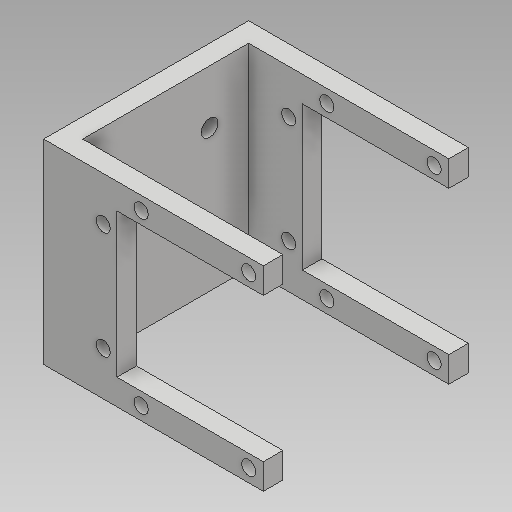
# Autodesk Inventor part: connection_hand
Saved by Autodesk Inventor 2017 (Build 210142000, 142)
## iProperties
Part Number: connection_hand
Material: Aluminium 6061
Document SubType Name: Modeling
Designer: Max
Density: 2.7 g/cm^3
Appearance: Vorgabe
Mass: 33.2037 g
Surface Area: 85.4905 cm^2
Volume: 12.2977 cm^3
Author: Max
Autodesk Inventor part; units mm, degrees
ref_plane "YZ Plane" through (0, 0, 0) normal (1, 0, 0) x (0, 1, 0)
ref_plane "XZ Plane" through (0, 0, 0) normal (0, 1, 0) x (-1, 0, 0)
ref_plane "XY Plane" through (0, 0, 0) normal (0, 0, 1) x (1, 0, 0)
sketch "Skizze1" plane through (0, 0, 0) normal (1, 0, 0) x (0, 1, 0)
  line L0 (-21, 20) -> (21, 20)
  line L1 (21, 20) -> (21, -20)
  line L2 (21, -20) -> (-21, -20)
  line L3 (-21, -20) -> (-21, 20)
  line L4 (-21, 20) -> (21, -20) construction
  line L5 (21, 20) -> (-21, -20) construction
  point P0 (0, 0)
  dimension "d0" = 42
  dimension "d1" = 40
  constraints: 12 end point, 2 midpoint, 2 parallel, 1 horizontal, 1 perpendicular
  measures "d0" distance of L1.end L2.end
  measures "d1" distance of L0.end L1.end
extrude "Extrusion1" add sketch "Skizze1" along normal blind 45
sketch "Skizze2" plane through (0, -21, 20) normal (0, 0, 1) x (1, 0, 0)
  line L0 (0, 0) -> (0, 42) projected
  line L1 (0, 0) -> (45, 0) projected
  line L2 (45, 42) -> (45, 0) projected
  line L3 (0, 42) -> (45, 42) projected
  line L4 (45, 42) -> (45, 0) projected
  line L5 (45, 38) -> (4, 38)
  line L6 (4, 38) -> (4, 4)
  line L7 (4, 4) -> (45, 4)
  line L8 (45, 4) -> (45, 38)
  point P0 (0, 21)
  dimension "d4" = 4
  dimension "d5" = 4
  dimension "d6" = 4
  constraints: 8 end point, 2 parallel, 1 horizontal, 1 perpendicular, 1 point on line
  measures "d4" distance between parallel lines of L5 L3
  measures "d5" distance between parallel lines of L1 L7
  measures "d6" distance between parallel lines of L0 L6
extrude "Extrusion2" cut sketch "Skizze2" against normal through all contours L7 L6 L5 L2
sketch "Skizze3" plane through (0, -21, -20) normal (0, -1, 0) x (1, 0, 0)
  line L0 (0, 0) -> (0, 40) projected
  line L1 (0, 0) -> (45, 0) projected
  line L2 (45, 40) -> (45, 0) projected
  line L3 (0, 40) -> (45, 40) projected
  line L4 (0, 20) -> (44.7617, 20) construction
  line L5 (15, 34.75) -> (45, 34.75)
  line L6 (45, 34.75) -> (45, 5.25)
  line L7 (45, 5.25) -> (15, 5.25)
  line L8 (15, 5.25) -> (15, 34.75)
  line L9 (15, 34.75) -> (45, 5.25) construction
  line L10 (45, 34.75) -> (15, 5.25) construction
  point P0 (30, 20)
  dimension "d9" = 29.5
  dimension "d10" = 30
  constraints: 14 end point, 2 horizontal, 2 midpoint, 2 parallel, 2 point on line, 1 perpendicular
  measures "d9" distance of L7.end L5.start
  measures "d10" distance of L6.end L7.end
extrude "Extrusion3" cut sketch "Skizze3" against normal through all contours L7 L8 L5 L2
sketch "Skizze4" plane through (0, -21, -20) normal (0, -1, 0) x (1, 0, 0)
  line L0 (45, 5.25) -> (15, 5.25) projected
  line L1 (15, 5.25) -> (15, 34.75) projected
  line L2 (15, 34.75) -> (45, 34.75) projected
  line L3 (45, 40) -> (45, 34.75) projected
  line L4 (0, 40) -> (45, 40) projected
  line L5 (0, 0) -> (0, 40) projected
  line L6 (0, 0) -> (45, 0) projected
  line L7 (45, 5.25) -> (45, 0) projected
  line L8 (0, 20) -> (84.4351, 20) construction
  point P0 (20, 37.3)
  point P1 (20, 2.7)
  point P2 (12.2, 31)
  point P3 (12.2, 9)
  point P4 (42, 37.3)
  point P5 (42, 2.7)
  dimension "d13" = 5
  dimension "d14" = 5
  dimension "d15" = 34.6
  dimension "d16" = 17.3
  dimension "d17" = 22
  dimension "d18" = 11
  dimension "d19" = 2.8
  dimension "d20" = 2.8
  dimension "d47" = 17.3
  dimension "d48" = 17.3
  dimension "d49" = 22
  dimension "d50" = 22
  constraints: 2 end point, 1 horizontal
  measures "d13" distance from line of point (20, 2.7) L1
  measures "d14" distance from line of L1 point (20, 37.3)
  measures "d15" distance of point (20, 2.7) point (20, 37.3)
  measures "d16" distance from line of L8 point (20, 37.3)
  measures "d17" distance of point (12.2, 9) point (12.2, 31)
  measures "d18" distance from line of L8 point (12.2, 31)
  measures "d19" distance from line of L1 point (12.2, 31)
  measures "d20" distance from line of L1 point (12.2, 9)
  measures "d47" distance from line of point (42, 37.3) L8
  measures "d48" distance from line of L8 point (42, 2.7)
  measures "d49" distance of point (42, 37.3) point (20, 37.3)
  measures "d50" distance of point (42, 2.7) point (20, 2.7)
hole "Bohrung1" at (20, -21, 17.3) at (20, -21, -17.3) at (12.2, -21, 11) at (12.2, -21, -11) at (42, -21, 17.3) at (42, -21, -17.3) direction (0, 1, 0) diameter 2.9 end through all clearance for "Inbusschraube ISO 4762" size "M2.5" standard "ISO"
sketch "Skizze7" plane through (4, -17, 20) normal (1, 0, 0) x (0, 0, -1)
  line L0 (29, 8) -> (11, 8)
  line L1 (11, 8) -> (11, 26)
  line L2 (11, 26) -> (29, 26)
  line L3 (29, 26) -> (29, 8)
  line L4 (29, 8) -> (11, 26) construction
  line L5 (11, 8) -> (29, 26) construction
  point P0 (20, 17)
  dimension "d52" = 18
  dimension "d53" = 18
  constraints: 12 end point, 2 midpoint, 2 parallel, 1 horizontal, 1 perpendicular
  measures "d52" distance of L1.end L2.end
  measures "d53" distance of L0.end L1.end
hole "Bohrung3" at (4, -9, 9) at (4, 9, 9) at (4, 9, -9) at (4, -9, -9) direction (-1, 0, 0) diameter 3.4 end through all clearance for "Inbusschraube ISO 4762" size "M3" standard "ISO"
equation "\"d5\" = d4"
equation "\"d13\" = d14"
equation "\"d16\" = 0.5 * d15"
equation "\"d18\" = 0.5 * d17"
equation "\"d20\" = d19"
equation "\"d47\" = d16"
equation "\"d48\" = d16"
equation "\"d50\" = d49"
equation "\"d53\" = d52"
